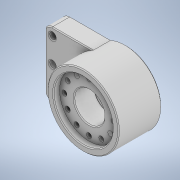
# Autodesk Inventor part: BearingStandoff2Falcon
Saved by Autodesk Inventor 2020 (Build 240168000, 168)
## iProperties
Created: 2020-02-02
Part Number: BearingStandoff2Falcon
Material: Generic
Document SubType Name: Modeling
Designer: srini
Density: 1 g/cm^3
Appearance: Default
Author: srini
Autodesk Inventor part; units mm, degrees
ref_plane "YZ Plane" through (0, 0, 0) normal (1, 0, 0) x (0, 1, 0)
ref_plane "XZ Plane" through (0, 0, 0) normal (0, 1, 0) x (-1, 0, 0)
ref_plane "XY Plane" through (0, 0, 0) normal (0, 0, 1) x (1, 0, 0)
sketch "Sketch1" plane through (0, 0, 0) normal (0, 0, 1) x (1, 0, 0)
  circle A0 centre (0, 0) radius 14.3002
  circle A1 centre (-57.15, 25.4) radius 3.3734
  line L0 (-57.15, 25.4) -> (-57.15, 19.7374)
  line L1 (-65.2734, 33.5234) -> (20.6502, 33.5234)
  line L2 (20.6502, 33.5234) -> (20.6502, -33.5234)
  line L3 (20.6502, -33.5234) -> (-65.2734, -33.5234)
  line L4 (-65.2734, -33.5234) -> (-65.2734, 33.5234)
  circle A2 centre (-57.15, 0) radius 3.3734
  line L5 (-57.15, 0) -> (-57.15, -5.6626)
  circle A3 centre (-57.15, -25.4) radius 3.3734
  line L6 (-57.15, -25.4) -> (-57.15, -31.0626)
  circle A4 centre (0, 0) radius 20.6502
  line L7 (-4.3196, 33.5234) -> (14.6019, 14.6019)
  line L8 (-4.3196, -33.5234) -> (14.6019, -14.6019)
  line L9 (-20.6502, 14.3879) -> (-20.6502, -18.7109) construction
  circle A5 centre (0, 0) radius 15.5575 construction
  line L10 (-15.5575, 17.5538) -> (-15.5575, -20.664) construction
  line L11 (-65.2734, 26.8016) -> (-66.675, 25.4)
  line L12 (-66.675, 25.4) -> (-66.675, -25.4)
  line L13 (-66.675, -25.4) -> (-65.2734, -26.8016)
  line L14 (-65.2734, -26.8016) -> (-65.2734, 26.8016)
  circle A6 centre (0, 0) radius 25.4 construction
  circle A7 centre (0, 0) radius 30.48
  circle A8 centre (0, 0) radius 36.83
  point P0 (-15.2521, -33.5234)
  point P1 (-15.2521, 33.5234)
  dimension "d0" = 28.6004
  dimension "d1" = 25.4
  dimension "d2" = 6.7469
  dimension "d6" = 25.4
  dimension "d11" = 8.1234
  dimension "d12" = 8.1234
  dimension "d13" = 8.1234
  dimension "d14" = 20.6502
  dimension "d15" = 45
  dimension "d16" = 45
  dimension "d43" = 31.115
  dimension "d45" = 57.15
  dimension "d46" = 41.5925
  dimension "d47" = 50.8
  dimension "d48" = 25.4
  dimension "d49" = 135
  dimension "d50" = 9.525
  dimension "d54" = 50.8
  dimension "d55" = 60.96
  dimension "d56" = 6.35
  constraints: 30 end point, 9 centre point, 6 coincident, 5 tangent, 5 vertical, 2 parallel, 2 perpendicular, 2 point on circle, 2 point on line, 1 collinear, 1 horizontal, 8 other
  measures "d0" diameter of A0
  measures "d1" vertical distance of L0.start point (0, 0)
  measures "d2" diameter of A1
  measures "d6" distance of L0.start L5.start
  measures "d11" distance from line of L0.start L1
  measures "d12" distance from line of L3 L6.start
  measures "d13" distance from line of L4 L0.start
  measures "d14" distance from line of L2 A0.centre
  measures "d15" angle of L7 L1
  measures "d16" angle of L3 L8
  measures "d43" diameter of A5
  measures "d45" horizontal distance of point (0, 0) L0.start
  measures "d46" distance from line of L5.start L10
  measures "d47" distance of L11.end L12.end
  measures "d48" vertical distance of L11.end point (0, 0)
  measures "d49" angle of L12 L11
  measures "d50" distance from line of L12 L5.start
  measures "d54" diameter of A6
  measures "d55" diameter of A7
  measures "d56" radial gap between concentric circles of A7 A8
extrude "Extrusion1" add sketch "Sketch1" along normal blind 19.05 contours L1 A8 L3 L4 | A8 L1 | L1 L7 A7 L8 L3 A8 | L4 L13 L12 L11 | L1 A8 L2 A7 L7 | L3 A8 | A7 L2 A4 L7 | L7 A4 L8 A7 | A8 L2 A7 | L8 A7 L2 A8 L3 | A4 | A7 L2 | L8 A4 L2 A7
fillet "Fillet1" radius 8.1234 2 edges at (-65.2734, -33.5234, 9.525) (-65.2734, 33.5234, 9.525)
sketch "Sketch2" plane through (0, 0, 19.05) normal (0, 0, 1) x (1, 0, 0)
  circle A0 centre (-9.0233, 15.6289) radius 2.0193
  line L0 (0, 0) -> (6.2322, 0)
  circle A1 centre (-9.0234, -15.6289) radius 2.0193
  circle A2 centre (18.0467, 0) radius 2.0193
  dimension "d20" = 18.0467
  dimension "d21" = 4.0386
  dimension "d22" = 120
  dimension "d25" = 360
  constraints: 3 centre point, 2 end point, 1 horizontal, 7 other
  measures "d20" distance of L0.start A0.centre
  measures "d21" diameter of A0
extrude "Extrusion2" [suppressed]
sketch "Sketch3" plane through (0, 0, 19.05) normal (0, 0, 1) x (1, 0, 0)
  circle A0 centre (0, 0) radius 15.5702
  dimension "d29" = 31.1404
  constraints: 1 centre point, 1 coincident
  measures "d29" diameter of A0
extrude "Extrusion3" cut sketch "Sketch3" against normal blind 1.6256
sketch "Sketch4" plane through (0, 0, 0) normal (0, 0, -1) x (-1, 0, 0)
  circle A0 centre (0, 0) radius 15.5702
  dimension "d32" = 31.1404
  constraints: 1 centre point, 1 coincident
  measures "d32" diameter of A0
extrude "Extrusion4" cut sketch "Sketch4" against normal blind 1.6256
chamfer "Chamfer1" distance 0.889 angle 45 16 edges at (-36.262, 33.5234, 19.05) (-62.497, 31.62, 19.05) (-62.497, -31.62, 19.05) (-36.262, -33.5234, 19.05) (-60.5234, 25.4, 19.05) (-60.5234, 0, 19.05) (-60.5234, -25.4, 19.05) (-14.3002, 0, 17.4244) (-14.3002, 0, 1.6256) (-60.5234, 25.4, 0) (-60.5234, 0, 0) (-60.5234, -25.4, 0) (-36.262, 33.5234, 0) (-62.497, 31.62, 0) (-62.497, -31.62, 0) (-36.262, -33.5234, 0)
chamfer "Chamfer2" distance 3.175 angle 45 2 edges at (-66.675, 0, 19.05) (-66.675, 0, 0)
sketch "Sketch6" plane through (0, 0, 19.05) normal (0, 0, 1) x (1, 0, 0)
  circle A0 centre (0, 25.4) radius 2.5797
  circle A1 centre (-12.7, 21.997) radius 2.5797
  circle A2 centre (-21.997, 12.7) radius 2.5797
  circle A3 centre (-25.4, 0) radius 2.5797
  circle A4 centre (-21.997, -12.7) radius 2.5797
  circle A5 centre (-12.7, -21.997) radius 2.5797
  circle A6 centre (0, -25.4) radius 2.5797
  circle A7 centre (12.7, -21.997) radius 2.5797
  circle A8 centre (21.997, -12.7) radius 2.5797
  circle A9 centre (25.4, 0) radius 2.5797
  circle A10 centre (21.997, 12.7) radius 2.5797
  circle A11 centre (12.7, 21.997) radius 2.5797
  point P0 (0, 0)
  dimension "d57" = 25.4
  dimension "d58" = 5.1594
  dimension "d61" = 360
  constraints: 12 centre point, 1 vertical alignment, 25 other
  measures "d57" distance of point (0, 0) A0.centre
  measures "d58" diameter of A0
extrude "Extrusion5" cut sketch "Sketch6" against normal through all
sketch "Sketch7" plane through (0, 0, 19.05) normal (0, 0, 1) x (1, 0, 0)
  circle A0 centre (-21.997, 12.7) radius 2.5797 projected
  circle A1 centre (21.997, -12.7) radius 2.5797 projected
  circle A2 centre (21.997, 12.7) radius 2.5797 projected
  circle A3 centre (-12.7, 21.997) radius 2.5797 projected
  circle A4 centre (-21.997, -12.7) radius 2.5797 projected
  circle A5 centre (25.4, 0) radius 2.5797 projected
  circle A6 centre (-12.7, -21.997) radius 2.5797 projected
  circle A7 centre (-25.4, 0) radius 2.5797 projected
  circle A8 centre (0, 25.4) radius 2.5797 projected
  circle A9 centre (12.7, -21.997) radius 2.5797 projected
  circle A10 centre (0, -25.4) radius 2.5797 projected
  circle A11 centre (12.7, 21.997) radius 2.5797 projected
  circle A12 centre (-57.15, -25.4) radius 4.2624 projected
  circle A13 centre (-57.15, 25.4) radius 4.2624 projected
  line L0 (-63.5, -29.0806) -> (-63.5, 29.0806) projected
  arc A14 (-63.5, -29.0806) -> (-57.2718, -32.6344) centre (-57.2718, -25.4) ccw projected
  line L1 (-17.0717, -32.6344) -> (-57.2718, -32.6344) projected
  arc A15 (-17.0717, -32.6344) -> (-17.0717, 32.6344) centre (0, 0) ccw projected
  line L2 (-57.2718, 32.6344) -> (-17.0717, 32.6344) projected
  arc A16 (-57.2718, 32.6344) -> (-63.5, 29.0806) centre (-57.2718, 25.4) ccw projected
  circle A17 centre (0, 0) radius 15.5702 projected
  circle A18 centre (-57.15, 0) radius 4.2624 projected
  circle A19 centre (0, 0) radius 14.3002 projected
  circle A20 centre (0, 0) radius 36.83
  point P0 (-17.0717, 32.6344)
  constraints: 1 centre point, 1 coincident, 1 concentric
extrude "Extrusion6" add sketch "Sketch7" along normal blind 19.05 contours A20 A15
sketch "Sketch8" plane through (0, 0, 38.1) normal (0, 0, 1) x (1, 0, 0)
  circle A0 centre (0, 0) radius 30.48
  circle A1 centre (0, 0) radius 36.83 projected
  dimension "d67" = 60.96
  constraints: 1 centre point, 1 coincident
  measures "d67" diameter of A0
extrude "Extrusion7" add sketch "Sketch8" along normal blind 6.35
sketch "Sketch9" plane through (0, 0, 0) normal (0, 0, -1) x (-1, 0, 0)
  circle A0 centre (-25.4, 0) radius 2.5797 projected
  circle A1 centre (-25.4, 0) radius 5.08
  circle A2 centre (-21.997, -12.7) radius 5.08
  circle A3 centre (-12.7, -21.997) radius 5.08
  circle A4 centre (0, -25.4) radius 5.08
  circle A5 centre (12.7, -21.997) radius 5.08
  circle A6 centre (21.997, -12.7) radius 5.08
  circle A7 centre (25.4, 0) radius 5.08
  circle A8 centre (21.997, 12.7) radius 5.08
  circle A9 centre (12.7, 21.997) radius 5.08
  circle A10 centre (0, 25.4) radius 5.08
  circle A11 centre (-12.7, 21.997) radius 5.08
  circle A12 centre (-21.997, 12.7) radius 5.08
  point P0 (0, 0)
  dimension "d70" = 10.16
  dimension "d73" = 360
  constraints: 12 centre point, 1 coincident, 25 other
  measures "d70" diameter of A1
extrude "Extrusion8" cut sketch "Sketch9" against normal blind 17.78 contours A0 | A1 | A2 | A3 | A4 | A5 | A6 | A7 | A8 | A9 | A10 | A11 | A12
sketch "Sketch10" plane through (25.4, 0, 17.78) normal (0, 0, -1) x (-1, 0, 0)
  line L0 (5.08, -2.5797) -> (-5.08, -2.5797)
  line L1 (-5.08, -2.5797) -> (-5.08, 2.5797)
  line L2 (-5.08, 2.5797) -> (5.08, 2.5797)
  line L3 (5.08, 2.5797) -> (5.08, -2.5797)
  circle A0 centre (0, 0) radius 2.5797 projected
  line L4 (5.08, -2.5797) -> (-5.08, 2.5797) construction
  line L5 (-5.08, -2.5797) -> (5.08, 2.5797) construction
  circle A1 centre (0, 0) radius 5.08 construction
  circle A2 centre (0, 0) radius 2.5797 projected
  line L6 (9.0922, -12.3941) -> (0.2934, -17.4741)
  line L7 (0.2934, -17.4741) -> (-2.2863, -13.0059)
  line L8 (-2.2863, -13.0059) -> (6.5125, -7.9259)
  line L9 (6.5125, -7.9259) -> (9.0922, -12.3941)
  line L10 (9.0922, -12.3941) -> (-2.2863, -13.0059) construction
  line L11 (0.2934, -17.4741) -> (6.5125, -7.9259) construction
  line L12 (17.4741, -18.8875) -> (12.3941, -27.6863)
  line L13 (12.3941, -27.6863) -> (7.9259, -25.1066)
  line L14 (7.9259, -25.1066) -> (13.0059, -16.3078)
  line L15 (13.0059, -16.3078) -> (17.4741, -18.8875)
  line L16 (17.4741, -18.8875) -> (7.9259, -25.1066) construction
  line L17 (12.3941, -27.6863) -> (13.0059, -16.3078) construction
  line L18 (27.9797, -20.32) -> (27.9797, -30.48)
  line L19 (27.9797, -30.48) -> (22.8203, -30.48)
  line L20 (22.8203, -30.48) -> (22.8203, -20.32)
  line L21 (22.8203, -20.32) -> (27.9797, -20.32)
  line L22 (27.9797, -20.32) -> (22.8203, -30.48) construction
  line L23 (27.9797, -30.48) -> (22.8203, -20.32) construction
  line L24 (37.7941, -16.3078) -> (42.8741, -25.1066)
  line L25 (42.8741, -25.1066) -> (38.4059, -27.6863)
  line L26 (38.4059, -27.6863) -> (33.3259, -18.8875)
  line L27 (33.3259, -18.8875) -> (37.7941, -16.3078)
  line L28 (37.7941, -16.3078) -> (38.4059, -27.6863) construction
  line L29 (42.8741, -25.1066) -> (33.3259, -18.8875) construction
  line L30 (44.2875, -7.9259) -> (53.0863, -13.0059)
  line L31 (53.0863, -13.0059) -> (50.5066, -17.4741)
  line L32 (50.5066, -17.4741) -> (41.7078, -12.3941)
  line L33 (41.7078, -12.3941) -> (44.2875, -7.9259)
  line L34 (44.2875, -7.9259) -> (50.5066, -17.4741) construction
  line L35 (53.0863, -13.0059) -> (41.7078, -12.3941) construction
  line L36 (45.72, 2.5797) -> (55.88, 2.5797)
  line L37 (55.88, 2.5797) -> (55.88, -2.5797)
  line L38 (55.88, -2.5797) -> (45.72, -2.5797)
  line L39 (45.72, -2.5797) -> (45.72, 2.5797)
  line L40 (45.72, 2.5797) -> (55.88, -2.5797) construction
  line L41 (55.88, 2.5797) -> (45.72, -2.5797) construction
  line L42 (41.7078, 12.3941) -> (50.5066, 17.4741)
  line L43 (50.5066, 17.4741) -> (53.0863, 13.0059)
  line L44 (53.0863, 13.0059) -> (44.2875, 7.9259)
  line L45 (44.2875, 7.9259) -> (41.7078, 12.3941)
  line L46 (41.7078, 12.3941) -> (53.0863, 13.0059) construction
  line L47 (50.5066, 17.4741) -> (44.2875, 7.9259) construction
  line L48 (33.3259, 18.8875) -> (38.4059, 27.6863)
  line L49 (38.4059, 27.6863) -> (42.8741, 25.1066)
  line L50 (42.8741, 25.1066) -> (37.7941, 16.3078)
  line L51 (37.7941, 16.3078) -> (33.3259, 18.8875)
  line L52 (33.3259, 18.8875) -> (42.8741, 25.1066) construction
  line L53 (38.4059, 27.6863) -> (37.7941, 16.3078) construction
  line L54 (22.8203, 20.32) -> (22.8203, 30.48)
  line L55 (22.8203, 30.48) -> (27.9797, 30.48)
  line L56 (27.9797, 30.48) -> (27.9797, 20.32)
  line L57 (27.9797, 20.32) -> (22.8203, 20.32)
  line L58 (22.8203, 20.32) -> (27.9797, 30.48) construction
  line L59 (22.8203, 30.48) -> (27.9797, 20.32) construction
  line L60 (13.0059, 16.3078) -> (7.9259, 25.1066)
  line L61 (7.9259, 25.1066) -> (12.3941, 27.6863)
  line L62 (12.3941, 27.6863) -> (17.4741, 18.8875)
  line L63 (17.4741, 18.8875) -> (13.0059, 16.3078)
  line L64 (13.0059, 16.3078) -> (12.3941, 27.6863) construction
  line L65 (7.9259, 25.1066) -> (17.4741, 18.8875) construction
  line L66 (6.5125, 7.9259) -> (-2.2863, 13.0059)
  line L67 (-2.2863, 13.0059) -> (0.2934, 17.4741)
  line L68 (0.2934, 17.4741) -> (9.0922, 12.3941)
  line L69 (9.0922, 12.3941) -> (6.5125, 7.9259)
  line L70 (6.5125, 7.9259) -> (0.2934, 17.4741) construction
  line L71 (-2.2863, 13.0059) -> (9.0922, 12.3941) construction
  point P0 (25.4, 0)
  point P1 (3.403, -12.7)
  point P2 (12.7, -21.997)
  point P3 (25.4, -25.4)
  point P4 (38.1, -21.997)
  point P5 (47.397, -12.7)
  point P6 (4.3763, 2.5797)
  point P7 (-4.3763, 2.5797)
  point P8 (-4.3763, -2.5797)
  point P9 (4.3763, -2.5797)
  point P10 (50.8, 0)
  point P11 (47.397, 12.7)
  point P12 (38.1, 21.997)
  point P13 (25.4, 25.4)
  point P14 (12.7, 21.997)
  point P15 (3.403, 12.7)
  dimension "d79" = 360
  constraints: 144 end point, 24 midpoint, 2 parallel, 2 tangent, 1 horizontal, 1 perpendicular, 133 other
extrude "Extrusion9" cut sketch "Sketch10" against normal blind 0.3
sketch "Sketch11" plane through (0, 0, 17.78) normal (0, 0, -1) x (-1, 0, 0)
  line L0 (-22.8203, -2.5797) -> (-27.9797, -2.5797)
  line L1 (-27.9797, -2.5797) -> (-27.9797, 2.5797)
  line L2 (-27.9797, 2.5797) -> (-22.8203, 2.5797)
  line L3 (-22.8203, 2.5797) -> (-22.8203, -2.5797)
  circle A0 centre (-25.4, 0) radius 2.5797 construction
  line L4 (-22.8203, -2.5797) -> (-27.9797, 2.5797) construction
  line L5 (-27.9797, -2.5797) -> (-22.8203, 2.5797) construction
  line L6 (-18.4731, -13.6442) -> (-22.9413, -16.2239)
  line L7 (-22.9413, -16.2239) -> (-25.521, -11.7558)
  line L8 (-25.521, -11.7558) -> (-21.0528, -9.1761)
  line L9 (-21.0528, -9.1761) -> (-18.4731, -13.6442)
  line L10 (-18.4731, -13.6442) -> (-25.521, -11.7558) construction
  line L11 (-22.9413, -16.2239) -> (-21.0528, -9.1761) construction
  line L12 (-9.1761, -21.0528) -> (-11.7558, -25.521)
  line L13 (-11.7558, -25.521) -> (-16.2239, -22.9413)
  line L14 (-16.2239, -22.9413) -> (-13.6442, -18.4731)
  line L15 (-13.6442, -18.4731) -> (-9.1761, -21.0528)
  line L16 (-9.1761, -21.0528) -> (-16.2239, -22.9413) construction
  line L17 (-11.7558, -25.521) -> (-13.6442, -18.4731) construction
  line L18 (2.5797, -22.8203) -> (2.5797, -27.9797)
  line L19 (2.5797, -27.9797) -> (-2.5797, -27.9797)
  line L20 (-2.5797, -27.9797) -> (-2.5797, -22.8203)
  line L21 (-2.5797, -22.8203) -> (2.5797, -22.8203)
  line L22 (2.5797, -22.8203) -> (-2.5797, -27.9797) construction
  line L23 (2.5797, -27.9797) -> (-2.5797, -22.8203) construction
  line L24 (13.6442, -18.4731) -> (16.2239, -22.9413)
  line L25 (16.2239, -22.9413) -> (11.7558, -25.521)
  line L26 (11.7558, -25.521) -> (9.1761, -21.0528)
  line L27 (9.1761, -21.0528) -> (13.6442, -18.4731)
  line L28 (13.6442, -18.4731) -> (11.7558, -25.521) construction
  line L29 (16.2239, -22.9413) -> (9.1761, -21.0528) construction
  line L30 (21.0528, -9.1761) -> (25.521, -11.7558)
  line L31 (25.521, -11.7558) -> (22.9413, -16.2239)
  line L32 (22.9413, -16.2239) -> (18.4731, -13.6442)
  line L33 (18.4731, -13.6442) -> (21.0528, -9.1761)
  line L34 (21.0528, -9.1761) -> (22.9413, -16.2239) construction
  line L35 (25.521, -11.7558) -> (18.4731, -13.6442) construction
  line L36 (22.8203, 2.5797) -> (27.9797, 2.5797)
  line L37 (27.9797, 2.5797) -> (27.9797, -2.5797)
  line L38 (27.9797, -2.5797) -> (22.8203, -2.5797)
  line L39 (22.8203, -2.5797) -> (22.8203, 2.5797)
  line L40 (22.8203, 2.5797) -> (27.9797, -2.5797) construction
  line L41 (27.9797, 2.5797) -> (22.8203, -2.5797) construction
  line L42 (18.4731, 13.6442) -> (22.9413, 16.2239)
  line L43 (22.9413, 16.2239) -> (25.521, 11.7558)
  line L44 (25.521, 11.7558) -> (21.0528, 9.1761)
  line L45 (21.0528, 9.1761) -> (18.4731, 13.6442)
  line L46 (18.4731, 13.6442) -> (25.521, 11.7558) construction
  line L47 (22.9413, 16.2239) -> (21.0528, 9.1761) construction
  line L48 (9.1761, 21.0528) -> (11.7558, 25.521)
  line L49 (11.7558, 25.521) -> (16.2239, 22.9413)
  line L50 (16.2239, 22.9413) -> (13.6442, 18.4731)
  line L51 (13.6442, 18.4731) -> (9.1761, 21.0528)
  line L52 (9.1761, 21.0528) -> (16.2239, 22.9413) construction
  line L53 (11.7558, 25.521) -> (13.6442, 18.4731) construction
  line L54 (-2.5797, 22.8203) -> (-2.5797, 27.9797)
  line L55 (-2.5797, 27.9797) -> (2.5797, 27.9797)
  line L56 (2.5797, 27.9797) -> (2.5797, 22.8203)
  line L57 (2.5797, 22.8203) -> (-2.5797, 22.8203)
  line L58 (-2.5797, 22.8203) -> (2.5797, 27.9797) construction
  line L59 (-2.5797, 27.9797) -> (2.5797, 22.8203) construction
  line L60 (-13.6442, 18.4731) -> (-16.2239, 22.9413)
  line L61 (-16.2239, 22.9413) -> (-11.7558, 25.521)
  line L62 (-11.7558, 25.521) -> (-9.1761, 21.0528)
  line L63 (-9.1761, 21.0528) -> (-13.6442, 18.4731)
  line L64 (-13.6442, 18.4731) -> (-11.7558, 25.521) construction
  line L65 (-16.2239, 22.9413) -> (-9.1761, 21.0528) construction
  line L66 (-21.0528, 9.1761) -> (-25.521, 11.7558)
  line L67 (-25.521, 11.7558) -> (-22.9413, 16.2239)
  line L68 (-22.9413, 16.2239) -> (-18.4731, 13.6442)
  line L69 (-18.4731, 13.6442) -> (-21.0528, 9.1761)
  line L70 (-21.0528, 9.1761) -> (-22.9413, 16.2239) construction
  line L71 (-25.521, 11.7558) -> (-18.4731, 13.6442) construction
  point P0 (0, 0)
  point P1 (-21.997, -12.7)
  point P2 (-12.7, -21.997)
  point P3 (0, -25.4)
  point P4 (12.7, -21.997)
  point P5 (21.997, -12.7)
  point P6 (25.4, 0)
  point P7 (21.997, 12.7)
  point P8 (12.7, 21.997)
  point P9 (0, 25.4)
  point P10 (-12.7, 21.997)
  point P11 (-21.997, 12.7)
  dimension "d85" = 360
  constraints: 144 end point, 24 midpoint, 2 parallel, 2 tangent, 1 horizontal, 1 perpendicular, 133 other
extrude "Extrusion10" cut sketch "Sketch11" against normal blind 0.6
chamfer "Chamfer3" distance 0.889 angle 45 4 edges at (36.83, 0, 0) (-36.83, 0, 44.45) (-30.48, 0, 44.45) (-15.5702, 0, 38.1)
equation "\"d12\" = d11"
equation "\"d13\" = d11"
equation "\"d48\" = 0.5 * d47"
equation "\"d19\" = d11"
body "Solid1"
